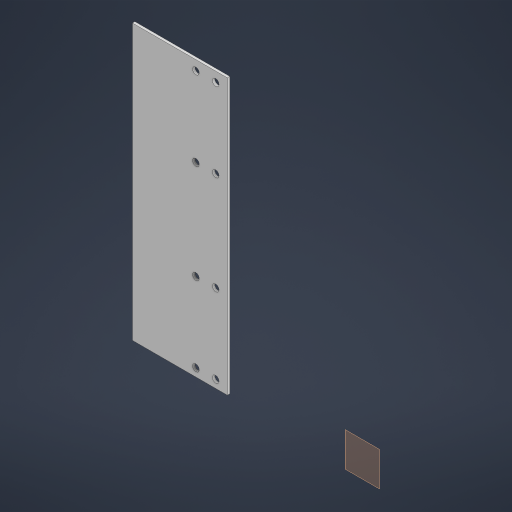
# Autodesk Inventor part: Horizontal wings poly
Saved by Autodesk Inventor 2023.4 (Build 274418000, 418)
## iProperties
Created: 2023-12-24
Part Number: Horizontal wings poly
Material: Generic
Document SubType Name: Modeling
Designer: diego
Density: 1 g/cm^3
Appearance: Default
Author: diego
Autodesk Inventor part; units mm, degrees
ref_plane "YZ Plane" through (0, 0, 0) normal (1, 0, 0) x (0, 1, 0)
ref_plane "XZ Plane" through (0, 0, 0) normal (0, 1, 0) x (-1, 0, 0)
ref_plane "XY Plane" through (0, 0, 0) normal (0, 0, 1) x (1, 0, 0)
ref_plane "Work Plane1" through (0, 0, 1.5875) normal (0, 0, 1) x (1, 0, 0)
sketch "Sketch2" plane through (0, 0, 1.5875) normal (0, 0, 1) x (1, 0, 0)
  line L0 (-85.1877, 170.4116) -> (-146.1477, 170.4116)
  line L1 (-146.1477, 170.4116) -> (-146.1477, -32.7884)
  line L2 (-146.1477, -32.7884) -> (-85.1877, -32.7884)
  line L3 (-85.1877, -32.7884) -> (-85.1877, 170.4116)
  circle A0 centre (-92.6614, 164.1359) radius 2.1844
  circle A1 centre (-92.6614, 151.4359) radius 2.1844
  circle A2 centre (-92.6614, 138.7359) radius 2.1844
  circle A3 centre (-92.6614, 126.0359) radius 2.1844
  circle A4 centre (-92.6614, -26.3641) radius 2.1844
  circle A5 centre (-92.6614, -13.6641) radius 2.1844
  circle A6 centre (-92.6614, -0.9641) radius 2.1844
  circle A7 centre (-92.6614, 11.7359) radius 2.1844
  circle A8 centre (-105.3614, 164.1359) radius 2.1844
  circle A9 centre (-105.3614, 151.4359) radius 2.1844
  circle A10 centre (-105.3614, 138.7359) radius 2.1844
  circle A11 centre (-105.3614, 126.0359) radius 2.1844
  circle A12 centre (-92.6614, 113.3359) radius 2.1844
  circle A13 centre (-105.3614, 113.3359) radius 2.1844
  circle A14 centre (-92.6614, 100.6359) radius 2.1844
  circle A15 centre (-105.3614, 100.6359) radius 2.1844
  circle A16 centre (-92.6614, 87.9359) radius 2.1844
  circle A17 centre (-105.3614, 87.9359) radius 2.1844
  circle A18 centre (-92.6614, 75.2359) radius 2.1844
  circle A19 centre (-105.3614, 75.2359) radius 2.1844
  circle A20 centre (-105.3614, -26.3641) radius 2.1844
  circle A21 centre (-105.3614, -13.6641) radius 2.1844
  circle A22 centre (-105.3614, -0.9641) radius 2.1844
  circle A23 centre (-105.3614, 11.7359) radius 2.1844
  circle A24 centre (-105.3614, 24.4359) radius 2.1844
  circle A25 centre (-105.3614, 37.1359) radius 2.1844
  circle A26 centre (-105.3614, 62.5359) radius 2.1844
  circle A27 centre (-105.3614, 49.8359) radius 2.1844
  circle A28 centre (-92.6614, 62.5359) radius 2.1844
  circle A29 centre (-92.6614, 49.8359) radius 2.1844
  line L4 (-90.858, 34.8245) -> (-94.4648, 34.8245)
  circle A30 centre (-92.6614, 24.4359) radius 2.1844
  circle A31 centre (-92.6614, 37.1359) radius 2.1844
  line L5 (-110.5377, 170.4116) -> (-110.5377, -32.7884)
  line L6 (-85.1877, -19.6806) -> (-146.1477, -19.6806)
  line L7 (-85.1877, -6.1071) -> (-146.1477, -6.1071)
  point P0 (0, 0)
  point P1 (-107.6728, 13.5393)
  dimension "d4" = 203.2
  dimension "d5" = 60.96
  constraints: 32 centre point, 16 end point, 6 point on line, 4 perpendicular, 2 parallel, 1 horizontal
  measures "d4" distance of L0.end L1.end
  measures "d5" distance of L1.end L2.end
extrude "Extrusion4" add sketch "Sketch2" along normal blind 1.5875 contours L3 L7 L5 L0 | L5 L7 L1 L0 | A1 | A2 | A3 | A7 | A9 | A10 | A11 | A14 | A15 | A16 | A17 | A18 | A19 | A23 | A24 | A25 | A26 | A28 | A30 | A31
body "Solid4"
